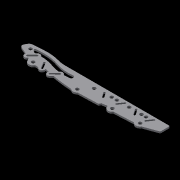
# Autodesk Inventor part: ForearmBaseLeft
Saved by Autodesk Inventor 2015 (Build 190159000, 159)
## iProperties
Created: 2014-10-05
Part Number: ForearmBaseLeft
Material: Generic
Document SubType Name: Modeling
Designer: Val
Density: 1 g/cm^3
Appearance: Default
Mass: 17.0012 g
Surface Area: 148.361 cm^2
Volume: 17.0012 cm^3
Author: Val
Autodesk Inventor part; units mm, degrees
ref_plane "YZ Plane" through (0, 0, 0) normal (1, 0, 0) x (0, 1, 0)
ref_plane "XZ Plane" through (0, 0, 0) normal (0, 1, 0) x (-1, 0, 0)
ref_plane "XY Plane" through (0, 0, 0) normal (0, 0, 1) x (1, 0, 0)
sketch "Base" plane through (0, 0, 0) normal (0, 0, 1) x (1, 0, 0)
  line L0 (-88.2296, 29.6083) -> (-106.7296, 28.2173)
  arc A0 (-106.7296, 28.2173) -> (-111.5, 25.1921) centre (-106.2797, 22.2342) ccw
  line L1 (-111.5, 25.1921) -> (-113.9649, 20.8419)
  arc A1 (-113.9649, 20.8419) -> (-111.808, 14.4812) centre (-110.0497, 18.6235) ccw
  line L2 (-111.808, 14.4812) -> (-98.6963, 8.9156)
  arc A2 (-98.6963, 8.9156) -> (-90.9909, 3.6412) centre (-94.3497, 7) ccw
  line L3 (-90.9909, 3.6412) -> (-90.0412, 4.591)
  arc A3 (-86.4745, -0.307) -> (-90.0412, 4.591) centre (-98.4774, -5.3) ccw
  arc A4 (-86.4745, -0.307) -> (-72.7826, -0.6602) centre (-79.5497, 2.5735) ccw
  arc A5 (-66.25, -1.7001) -> (-72.7826, -0.6602) centre (-71, -10.5) ccw
  arc A6 (-66.25, -1.7001) -> (-57.9832, 2.9682) centre (-62.2, 0.7817) ccw
  arc A7 (-57.9832, 2.9682) -> (-51.2774, 1.3823) centre (11.1884, 280.4773) ccw
  arc A8 (-51.2774, 1.3823) -> (-43.7004, -4.1001) centre (-47, -0.6832) ccw
  line L4 (-43.7004, -4.1001) -> (-40.3291, -0.8445)
  arc A9 (-40.3291, -0.8445) -> (-5.5616, -5.0318) centre (11.1884, 280.4773) ccw
  arc A10 (-59.3435, 26.7816) -> (-88.2296, 29.6083) centre (-81.8939, -54.6538) ccw
  arc A11 (-59.3435, 26.7816) -> (-46, 24.9682) centre (-46, 74.9682) ccw
  arc A12 (-5.5616, -5.0318) -> (5.6654, -4.9146) centre (0, 0) ccw
  line L5 (5.6654, -4.9146) -> (53.6654, -3.2384)
  arc A13 (53.6654, -3.2384) -> (65.7753, -2.6463) centre (59.5047, 1.4682) ccw
  line L6 (65.7753, -2.6463) -> (99.8785, -0.8584)
  arc A14 (99.8785, -0.8584) -> (112.3745, -0.491) centre (106.0047, 3.4682) ccw
  line L7 (112.3745, -0.491) -> (136.3745, 8.2153)
  line L8 (165.7955, 19.8419) -> (164.8009, 23.8311) construction
  arc A15 (165.1662, 18.6599) -> (165.7955, 19.8419) centre (164.8252, 19.6) ccw construction
  line L9 (-46, 24.9682) -> (136.3745, 24.9682)
  arc A16 (164.8009, 23.8311) -> (163.3454, 24.9682) centre (163.3454, 23.4682) ccw construction
  line L10 (136.3745, 8.2153) -> (136.3745, 24.9682)
  line L11 (136.3745, 24.9682) -> (163.3454, 24.9682) construction
  line L12 (136.3745, 8.2153) -> (165.1662, 18.6599) construction
  point P0 (164.5173, 24.9682)
  point P1 (-90.5161, 4.1161)
  dimension "d57" = 1.5
  dimension "d58" = 24
  constraints: 34 point on circle, 26 end point, 17 centre point, 4 horizontal, 3 tangent, 2 point on line, 1 midpoint, 1 vertical, 26 other
  measures "d57" radius of A16
  measures "d58" distance from line of L10 L7.start
extrude "BaseFeature" add sketch "Base" along normal blind 3
sketch "Rails" plane through (0, 0, 3) normal (0, 0, 1) x (1, 0, 0)
  circle A0 centre (72.3941, 17.9682) radius 2.4585 projected
  circle A1 centre (51.0047, 17.9682) radius 2.4585 projected
  circle A2 centre (42.0047, 17.9682) radius 2.4585 projected
  line L0 (112.4005, 21.3286) -> (106.0987, 12.3286) projected
  arc A3 (106.0987, 12.3286) -> (108.5561, 10.6079) centre (107.3274, 11.4682) ccw projected
  line L1 (108.5561, 10.6079) -> (114.858, 19.6079) projected
  arc A4 (114.858, 19.6079) -> (112.4005, 21.3286) centre (113.6293, 20.4682) ccw projected
  line L2 (89.4685, 12.3286) -> (83.1667, 21.3286) projected
  arc A5 (83.1667, 21.3286) -> (80.7092, 19.6079) centre (81.9379, 20.4682) ccw projected
  line L3 (80.7092, 19.6079) -> (87.0111, 10.6079) projected
  arc A6 (87.0111, 10.6079) -> (89.4685, 12.3286) centre (88.2398, 11.4682) ccw projected
  circle A7 centre (72.3941, 17.9682) radius 2.4585 projected
  line L4 (57.7772, 10.6079) -> (64.0791, 19.6079) projected
  arc A8 (64.0791, 19.6079) -> (61.6216, 21.3286) centre (62.8503, 20.4682) ccw projected
  line L5 (61.6216, 21.3286) -> (55.3198, 12.3286) projected
  arc A9 (55.3198, 12.3286) -> (57.7772, 10.6079) centre (56.5485, 11.4682) ccw projected
  circle A10 centre (134.0047, 23.9682) radius 1.2295 projected
  circle A11 centre (158.0047, 23.9682) radius 1.2295 projected
  circle A12 centre (72.3941, 17.9682) radius 2.4585 projected
  circle A13 centre (93.7836, 17.9682) radius 2.4585 projected
  circle A14 centre (101.7836, 17.9682) radius 2.4585 projected
  line L6 (-39.0502, 9.079) -> (-48.042, 0.3958) projected
  arc A15 (-36.9663, 6.921) -> (-39.0502, 9.079) centre (-38.0083, 8) ccw projected
  line L7 (-45.958, -1.7622) -> (-36.9663, 6.921) projected
  arc A16 (-48.042, 0.3958) -> (-45.958, -1.7622) centre (-47, -0.6832) ccw projected
  arc A17 (-63.479, -0.002) -> (-60.921, 1.5655) centre (-62.2, 0.7817) ccw projected
  line L8 (-60.921, 1.5655) -> (-67.4523, 12.2235) projected
  line L9 (-70.0102, 10.656) -> (-63.479, -0.002) projected
  arc A18 (-67.4523, 12.2235) -> (-70.0102, 10.656) centre (-68.7312, 11.4398) ccw projected
  line L10 (-93.289, 5.9393) -> (-84.4502, 14.7782) projected
  arc A19 (-84.4502, 14.7782) -> (-86.5715, 16.8995) centre (-85.5109, 15.8388) ccw projected
  line L11 (-86.5715, 16.8995) -> (-95.4104, 8.0607) projected
  arc A20 (-95.4104, 8.0607) -> (-93.289, 5.9393) centre (-94.3497, 7) ccw projected
  circle A21 centre (13.3989, 15.9682) radius 2.4585 projected
  line L12 (35.7615, 11.2239) -> (30.0865, 19.3286) projected
  arc A22 (33.304, 9.5031) -> (35.7615, 11.2239) centre (34.5328, 10.3635) ccw projected
  arc A23 (30.0865, 19.3286) -> (27.629, 17.6079) centre (28.8578, 18.4682) ccw projected
  line L13 (27.629, 17.6079) -> (33.304, 9.5031) projected
  line L14 (-95.4104, 8.0607) -> (-86.5715, 16.8995)
  arc A24 (-95.4104, 8.0607) -> (-93.289, 5.9393) centre (-94.3497, 7) ccw
  line L15 (-84.4502, 14.7782) -> (-93.289, 5.9393)
  arc A25 (-84.4502, 14.7782) -> (-86.5715, 16.8995) centre (-85.5109, 15.8388) ccw
  arc A26 (-67.4523, 12.2235) -> (-70.0102, 10.656) centre (-68.7312, 11.4398) ccw
  line L16 (-63.479, -0.002) -> (-70.0102, 10.656)
  line L17 (-67.4523, 12.2235) -> (-60.921, 1.5655)
  arc A27 (-63.479, -0.002) -> (-60.921, 1.5655) centre (-62.2, 0.7817) ccw
  line L18 (-48.042, 0.3958) -> (-39.0502, 9.079)
  arc A28 (-48.042, 0.3958) -> (-45.958, -1.7622) centre (-47, -0.6832) ccw
  line L19 (-36.9663, 6.921) -> (-45.958, -1.7622)
  arc A29 (-36.9663, 6.921) -> (-39.0502, 9.079) centre (-38.0083, 8) ccw
  line L20 (33.304, 9.5031) -> (27.629, 17.6079)
  arc A30 (30.0865, 19.3286) -> (27.629, 17.6079) centre (28.8578, 18.4682) ccw
  line L21 (30.0865, 19.3286) -> (35.7615, 11.2239)
  arc A31 (33.304, 9.5031) -> (35.7615, 11.2239) centre (34.5328, 10.3635) ccw
  arc A32 (55.3198, 12.3286) -> (57.7772, 10.6079) centre (56.5485, 11.4682) ccw
  line L22 (64.0791, 19.6079) -> (57.7772, 10.6079)
  line L23 (55.3198, 12.3286) -> (61.6216, 21.3286)
  arc A33 (64.0791, 19.6079) -> (61.6216, 21.3286) centre (62.8503, 20.4682) ccw
  arc A34 (83.1667, 21.3286) -> (80.7092, 19.6079) centre (81.9379, 20.4682) ccw
  line L24 (87.0111, 10.6079) -> (80.7092, 19.6079)
  line L25 (83.1667, 21.3286) -> (89.4685, 12.3286)
  arc A35 (87.0111, 10.6079) -> (89.4685, 12.3286) centre (88.2398, 11.4682) ccw
  line L26 (106.0987, 12.3286) -> (112.4005, 21.3286)
  arc A36 (114.858, 19.6079) -> (112.4005, 21.3286) centre (113.6293, 20.4682) ccw
  line L27 (114.858, 19.6079) -> (108.5561, 10.6079)
  arc A37 (106.0987, 12.3286) -> (108.5561, 10.6079) centre (107.3274, 11.4682) ccw
  arc A38 (-102.0167, 23.4581) -> (-101.0827, 16.5207) centre (-101.5497, 19.9894) ccw construction
  spline S0 degree 3 poles (-20.9034, 11.8689) (-20.699, 12.2669) (-20.5753, 12.705) (-20.4895, 13.5682) (-20.5334, 14.0463) (-20.8057, 14.9369) (-21.0336, 15.3499) (-21.5235, 15.9479) (-21.7901, 16.193) (-22.0935, 16.3926) knots 0.402356 0.402356 0.402356 0.402356 0.529128 0.529128 0.66478 0.66478 0.800432 0.800432 0.906058 0.906058 0.906058 0.906058
  arc A39 (-55.7151, 20.4123) -> (-24.4179, 16.9452) centre (-32.5, 86.9804) ccw
  arc A40 (-22.0935, 16.3926) -> (-24.4179, 16.9452) centre (-24.0166, 13.4682) ccw
  arc A41 (-55.7151, 20.4123) -> (-82.5497, 24.8435) centre (-81.8939, -54.6538) ccw
  arc A42 (-82.5497, 24.8435) -> (-98.0321, 23.9424) centre (-81.267, -130.6512) ccw
  spline S1 degree 3 poles (-102.0167, 23.4581) (-102.2026, 23.4331) (-102.3877, 23.3929) (-103.0138, 23.2025) (-103.4291, 22.9741) (-104.1043, 22.4214) (-104.4106, 22.059) (-104.8528, 21.2372) (-104.9886, 20.7776) (-105.0359, 20.302) (-105.0388, 20.268) (-105.0412, 20.2339) knots -0.985233 -0.985233 -0.985233 -0.985233 -0.931443 -0.931443 -0.798305 -0.798305 -0.665074 -0.665074 -0.531843 -0.531843 -0.52167 -0.52167 -0.52167 -0.52167 construction
  arc A43 (-90.5061, 17.5611) -> (-101.0827, 16.5207) centre (-81.267, -130.6512) ccw construction
  arc A44 (-58.0202, 13.8027) -> (-81.2043, 17.8429) centre (-81.8939, -54.6538) ccw
  arc A45 (-58.0202, 13.8027) -> (-42.6253, 10.1446) centre (-32.5, 86.9804) ccw
  arc A46 (-33.4969, 9.4868) -> (-23.6154, 9.9913) centre (-32.5, 86.9804) ccw
  arc A47 (-58.0202, 13.8027) -> (-81.2043, 17.8429) centre (-81.8939, -54.6538) ccw
  arc A48 (-81.2043, 17.8429) -> (-88.8696, 19.1976) centre (-85.5109, 15.8388) ccw
  arc A49 (-33.4969, 9.4868) -> (-41.3079, 11.4169) centre (-38.0083, 8) ccw
  line L28 (-41.3079, 11.4169) -> (-42.6253, 10.1446)
  arc A50 (-23.6154, 9.9913) -> (-24.4179, 16.9452) centre (-24.0166, 13.4682) ccw
  line L29 (-88.8696, 19.1976) -> (-90.5061, 17.5611)
  arc A51 (-98.0321, 23.9424) -> (-90.5061, 17.5611) centre (-90.9491, 24.6673) ccw
  point P0 (0, 0)
  constraints: 56 point on circle, 32 end point, 28 centre point, 1 tangent, 119 other
sketch "RailsProjection" plane through (0, 0, 3) normal (0, 0, 1) x (1, 0, 0)
  arc A0 (-98.0321, 23.9424) -> (-90.5061, 17.5611) centre (-90.9491, 24.6673) ccw projected
  arc A1 (-82.5497, 24.8435) -> (-98.0321, 23.9424) centre (-81.267, -130.6512) ccw projected
  line L0 (-88.8696, 19.1976) -> (-90.5061, 17.5611) projected
  arc A2 (-81.2043, 17.8429) -> (-88.8696, 19.1976) centre (-85.5109, 15.8388) ccw projected
  arc A3 (-55.7151, 20.4123) -> (-82.5497, 24.8435) centre (-81.8939, -54.6538) ccw projected
  arc A4 (-58.0202, 13.8027) -> (-81.2043, 17.8429) centre (-81.8939, -54.6538) ccw projected
  arc A5 (-55.7151, 20.4123) -> (-24.4179, 16.9452) centre (-32.5, 86.9804) ccw projected
  arc A6 (-58.0202, 13.8027) -> (-42.6253, 10.1446) centre (-32.5, 86.9804) ccw projected
  line L1 (-41.3079, 11.4169) -> (-42.6253, 10.1446) projected
  arc A7 (-33.4969, 9.4868) -> (-41.3079, 11.4169) centre (-38.0083, 8) ccw projected
  arc A8 (-33.4969, 9.4868) -> (-23.6154, 9.9913) centre (-32.5, 86.9804) ccw projected
  arc A9 (-23.6154, 9.9913) -> (-24.4179, 16.9452) centre (-24.0166, 13.4682) ccw projected
  line L2 (-86.5715, 16.8995) -> (-95.4104, 8.0607) projected
  arc A10 (-84.4502, 14.7782) -> (-86.5715, 16.8995) centre (-85.5109, 15.8388) ccw projected
  line L3 (-93.289, 5.9393) -> (-84.4502, 14.7782) projected
  arc A11 (-95.4104, 8.0607) -> (-93.289, 5.9393) centre (-94.3497, 7) ccw projected
  arc A12 (-67.4523, 12.2235) -> (-70.0102, 10.656) centre (-68.7312, 11.4398) ccw projected
  line L4 (-70.0102, 10.656) -> (-63.479, -0.002) projected
  line L5 (-60.921, 1.5655) -> (-67.4523, 12.2235) projected
  arc A13 (-63.479, -0.002) -> (-60.921, 1.5655) centre (-62.2, 0.7817) ccw projected
  arc A14 (-48.042, 0.3958) -> (-45.958, -1.7622) centre (-47, -0.6832) ccw projected
  line L6 (-39.0502, 9.079) -> (-48.042, 0.3958) projected
  line L7 (-45.958, -1.7622) -> (-36.9663, 6.921) projected
  arc A15 (-36.9663, 6.921) -> (-39.0502, 9.079) centre (-38.0083, 8) ccw projected
  arc A16 (30.0865, 19.3286) -> (27.629, 17.6079) centre (28.8578, 18.4682) ccw projected
  line L8 (27.629, 17.6079) -> (33.304, 9.5031) projected
  line L9 (35.7615, 11.2239) -> (30.0865, 19.3286) projected
  arc A17 (33.304, 9.5031) -> (35.7615, 11.2239) centre (34.5328, 10.3635) ccw projected
  arc A18 (55.3198, 12.3286) -> (57.7772, 10.6079) centre (56.5485, 11.4682) ccw projected
  line L10 (61.6216, 21.3286) -> (55.3198, 12.3286) projected
  line L11 (57.7772, 10.6079) -> (64.0791, 19.6079) projected
  arc A19 (64.0791, 19.6079) -> (61.6216, 21.3286) centre (62.8503, 20.4682) ccw projected
  arc A20 (83.1667, 21.3286) -> (80.7092, 19.6079) centre (81.9379, 20.4682) ccw projected
  line L12 (80.7092, 19.6079) -> (87.0111, 10.6079) projected
  line L13 (83.1667, 21.3286) -> (89.4685, 12.3286) projected
  arc A21 (87.0111, 10.6079) -> (89.4685, 12.3286) centre (88.2398, 11.4682) ccw projected
  arc A22 (106.0987, 12.3286) -> (108.5561, 10.6079) centre (107.3274, 11.4682) ccw projected
  line L14 (112.4005, 21.3286) -> (106.0987, 12.3286) projected
  line L15 (108.5561, 10.6079) -> (114.858, 19.6079) projected
  arc A23 (114.858, 19.6079) -> (112.4005, 21.3286) centre (113.6293, 20.4682) ccw projected
  point P0 (0, 0)
extrude "RailsFeature" cut sketch "RailsProjection" against normal through all
sketch "BaseHoles" plane through (0, 0, 0) normal (0, 0, -1) x (-1, 0, 0)
  arc A0 (-112.3745, -0.491) -> (-99.8785, -0.8584) centre (-106.0047, 3.4682) ccw projected
  arc A1 (-65.7753, -2.6463) -> (-53.6654, -3.2384) centre (-59.5047, 1.4682) ccw projected
  arc A2 (72.7826, -0.6602) -> (86.4745, -0.307) centre (79.5497, 2.5735) ccw projected
  point P0 (0, 0)
hole "BaseHolesFeature" at (106.0047, 3.4682, 0) at (59.5047, 1.4682, 0) at (0, 0, 0) at (-79.5497, 2.5735, 0) direction (0, 0, 1) diameter 6 end through all
hole "TopHolesFeature" at (13.3989, 15.9682, 3) at (42.0047, 17.9682, 3) at (51.0047, 17.9682, 3) at (72.3941, 17.9682, 3) at (93.7836, 17.9682, 3) at (101.7836, 17.9682, 3) direction (0, 0, -1) diameter 6 end through all
hole "CableConnectorHoleFeature" at (-101.5497, 19.9894, 3) direction (0, 0, -1) diameter 6 end through all
fillet "LipFilletFeature" radius 1 1 edges at (-98.0321, 23.9424, 1.5)
sketch "BottomCut" plane through (0, 0, 3) normal (0, 0, 1) x (1, 0, 0)
  arc A0 (43.1539, -0.195) -> (50.842, 1.1334) centre (40, 40.9682) ccw construction
  arc A1 (52.0929, 0.3214) -> (50.842, 1.1334) centre (51.1046, 0.1685) ccw construction
  arc A2 (52.0929, 0.3214) -> (66.9872, 1.9798) centre (59.5047, 1.4682) ccw construction
  arc A3 (43.1539, -0.195) -> (50.842, 1.1334) centre (40, 40.9682) ccw construction
  arc A4 (43.1539, -0.195) -> (42.3315, -0.7537) centre (43.2303, -1.1921) ccw construction
  line L0 (41.1656, -3.1441) -> (42.3315, -0.7537) construction
  arc A5 (40.3017, -3.7051) -> (41.1656, -3.1441) centre (40.2668, -2.7057) ccw construction
  arc A6 (52.0929, 0.3214) -> (53.6654, -3.2384) centre (59.5047, 1.4682) ccw
  arc A7 (52.0929, 0.3214) -> (50.842, 1.1334) centre (51.1046, 0.1685) ccw
  arc A8 (40.3017, -3.7051) -> (41.1656, -3.1441) centre (40.2668, -2.7057) ccw
  line L1 (41.1656, -3.1441) -> (42.3315, -0.7537)
  arc A9 (43.1539, -0.195) -> (42.3315, -0.7537) centre (43.2303, -1.1921) ccw
  arc A10 (43.1539, -0.195) -> (50.842, 1.1334) centre (40, 40.9682) ccw
  line L2 (40.3017, -3.7051) -> (37.6613, -3.7973)
  line L3 (5.6654, -4.9146) -> (53.6654, -3.2384) construction
  line L4 (37.6613, -3.7973) -> (37.6613, -4.7973)
  line L5 (53.6654, -3.2384) -> (53.6654, -4.2384)
  line L6 (53.6654, -4.2384) -> (37.6613, -4.7973)
  dimension "d39" = 1
  constraints: 22 point on circle, 12 end point, 11 centre point, 5 tangent, 2 concentric, 2 parallel, 1 collinear, 1 point on line, 1 vertical, 20 other
  measures "d39" distance of L2.end L4.end
extrude "BottomCutFeature" cut sketch "BottomCut" against normal through all
fillet "BaseFilletsFeature" radius 2 2 edges at (136.3745, 24.9682, 1.5) (136.3745, 8.2153, 1.5)
